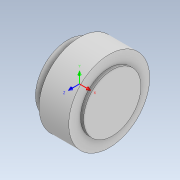
# Autodesk Inventor part: motor
Saved by Autodesk Inventor 2020 (Build 240168000, 168)
## iProperties
Created: 2021-01-12
Part Number: motor
Material: Generic
Document SubType Name: Modeling
Designer: DELL
Density: 1 g/cm^3
Appearance: Default
Author: DELL
Autodesk Inventor part; units mm, degrees
ref_plane "YZ Plane" through (0, 0, 0) normal (1, 0, 0) x (0, 1, 0)
ref_plane "XZ Plane" through (0, 0, 0) normal (0, 1, 0) x (-1, 0, 0)
ref_plane "XY Plane" through (0, 0, 0) normal (0, 0, 1) x (1, 0, 0)
sketch "Sketch1" plane through (0, 0, 0) normal (1, 0, 0) x (0, 1, 0)
  circle A0 centre (0, 0) radius 31.5
  circle A1 centre (0, 0) radius 39.5
  circle A2 centre (0, 0) radius 28
  dimension "d0" = 79
  dimension "d1" = 63
  dimension "d12" = 56
  constraints: 3 centre point, 3 coincident
  measures "d0" diameter of A1
  measures "d1" diameter of A0
  measures "d12" diameter of A2
extrude "Extrusion1" add sketch "Sketch1" against normal blind 11.5 contours A0 | A2
extrude "Extrusion2" add sketch "Sketch1" along normal blind 29 contours A0 | A1 | A2
extrude "Extrusion3" add sketch "Sketch1" along normal blind 3 from surface at 29 contours A2
body "Solid1"
